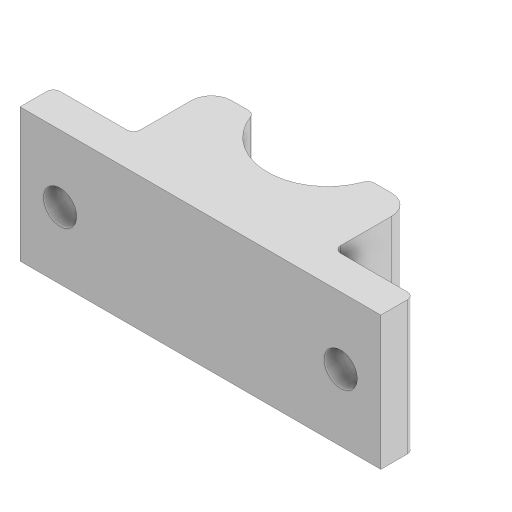
# Autodesk Inventor part: Shaft support
Saved by Autodesk Inventor 2023 (Build 270158000, 158)
## iProperties
Created: 2023-02-28
Part Number: Shaft support
Material: Generic
Document SubType Name: Modeling
Designer: david
Density: 1 g/cm^3
Appearance: Default
Author: david
Autodesk Inventor part; units mm, degrees
ref_plane "YZ Plane" through (0, 0, 0) normal (1, 0, 0) x (0, 1, 0)
ref_plane "XZ Plane" through (0, 0, 0) normal (0, 1, 0) x (-1, 0, 0)
ref_plane "XY Plane" through (0, 0, 0) normal (0, 0, 1) x (1, 0, 0)
sketch "Sketch1" plane through (0, 0, 0) normal (0, 1, 0) x (-1, 0, 0)
  circle A0 centre (0, -19.05) radius 9
  line L0 (15, 0) -> (-15, 0)
  line L1 (-15, 0) -> (-15, -16.6415)
  line L2 (-15, -16.6415) -> (15, -16.6415)
  line L3 (15, -16.6415) -> (15, 0)
  line L4 (-27, -5) -> (27, -5)
  line L5 (27, -5) -> (27, 0)
  line L6 (27, 0) -> (-27, 0)
  line L7 (-27, 0) -> (-27, -5)
  line L8 (-27, -5) -> (27, 0) construction
  line L9 (27, -5) -> (-27, 0) construction
  point P0 (0, 0)
  point P1 (0, -2.5)
  point P2 (0, -2.5)
  point P3 (0, -2.5)
  point P4 (15, -5)
  point P5 (15, 0)
  point P6 (-15, -5)
  point P7 (-15, 0)
  point P8 (0, 0)
  dimension "d0" = 18
  dimension "d1" = 19.05
  dimension "d5" = 15
  dimension "d6" = 15
  dimension "d7" = 27
  dimension "d13" = 5
  constraints: 20 end point, 7 midpoint, 4 parallel, 2 horizontal, 2 perpendicular, 2 vertical alignment, 1 centre point
  measures "d0" diameter of A0
  measures "d1" distance of point (0, 0) A0.centre
  measures "d5" distance from line of L1 A0.centre
  measures "d6" distance from line of L3 A0.centre
  measures "d7" distance from line of L7 point (0, -2.5)
  measures "d13" distance of L6.end L4.start
extrude "Extrusion1" add sketch "Sketch1" along normal blind 20 contours A0 L2 L1 L4 L3 | L4 L1 L0 L3 | L3 L6 L5 L4 | L4 L7 L6 L1
sketch "Sketch2" plane through (27, 0, -5) normal (0, 0, -1) x (-1, 0, 0)
  circle A0 centre (6, 10) radius 2.5
  line L0 (0, 0) -> (0, 20) projected
  line L1 (0, 20) -> (12, 20) projected
  point P0 (27, 0)
  point P1 (6, 20)
  dimension "d10" = 6
  dimension "d11" = 10
  dimension "d12" = 5
  constraints: 1 centre point, 1 midpoint
  measures "d10" distance from line of L0 A0.centre
  measures "d11" distance of point (6, 20) A0.centre
  measures "d12" diameter of A0
extrude "Extrusion2" cut sketch "Sketch2" against normal through all
mirror "Mirror1" about plane through (0, 0, 0) normal (1, 0, 0) of "Extrusion2"
fillet "Fillet2" radius 1 2 edges at (8.6718, 10, -16.6415) (-8.6718, 10, -16.6415)
fillet "Fillet3" radius 1 2 edges at (27, 10, -5) (-27, 10, -5)
sketch "Sketch3" plane through (-15, 0, -5) normal (0, 0, -1) x (-1, 0, 0)
  circle A0 centre (6, 10) radius 2.5 projected
  circle A1 centre (6, 10) radius 5
  line L0 (11, 20) -> (11, 0) projected
  point P0 (-15, 0)
  constraints: 1 centre point, 1 coincident, 1 tangent
fillet "Fillet4" radius 1 2 edges at (15, 10, -5) (-15, 10, -5)
fillet "Fillet5" radius 3 2 edges at (15, 10, -16.6415) (-15, 10, -16.6415)
body "Solid1"
